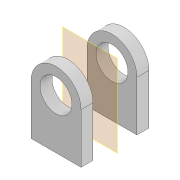
# Autodesk Inventor part: UnionMarco
Saved by Autodesk Inventor 2021 (Build 250183000, 183)
## iProperties
Created: 2021-05-08
Part Number: UnionMarco
Material: Generic
Document SubType Name: Modeling
Designer: Santiago Suárez
Density: 1 g/cm^3
Appearance: Default
Author: Santiago Suárez
Autodesk Inventor part; units mm, degrees
ref_plane "YZ Plane" through (0, 0, 0) normal (1, 0, 0) x (0, 1, 0)
ref_plane "XZ Plane" through (0, 0, 0) normal (0, 1, 0) x (-1, 0, 0)
ref_plane "XY Plane" through (0, 0, 0) normal (0, 0, 1) x (1, 0, 0)
sketch "Sketch1" plane through (0, 0, 0) normal (0, 0, 1) x (1, 0, 0)
  circle A0 centre (0, 0) radius 8
  arc A1 (12.5, 0) -> (-12.5, 0) centre (0, 0) ccw
  line L0 (-12.5, 0) -> (-12.5, -25)
  line L1 (12.5, 0) -> (12.5, -25)
  line L2 (-12.5, -25) -> (12.5, -25)
  dimension "d0" = 16
  dimension "d1" = 25
  dimension "d2" = 25
  dimension "d3" = 25
  constraints: 6 end point, 2 centre point, 2 coincident, 2 point on circle, 2 tangent, 2 vertical
  measures "d0" diameter of A0
  measures "d1" diameter of A1
  measures "d2" distance of L0.start L0.end
  measures "d3" distance of L1.start L1.end
extrude "Extrusion1" add sketch "Sketch1" along normal blind 6
ref_plane "Work Plane1" through (0, 0, 17) normal (0, 0, 1) x (1, 0, 0)
mirror "Mirror1" about plane through (0, 0, 17) normal (0, 0, 1) of "Extrusion1"
body "Solid1"
